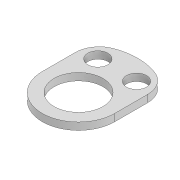
# Autodesk Inventor part: Sujeción mangueras
Saved by Autodesk Inventor 2022 (Build 260153000, 153)
## iProperties
Created: 2022-10-26
Part Number: Sujeción mangueras
Material: Generic
Document SubType Name: Modeling
Designer: ADMIN
Density: 1 g/cm^3
Appearance: Default
Author: ADMIN
## iProperties of the stored document Sujeción mangueras_3DPrint.ipt
Created: 2022-10-26
Part Number: Sujeción mangueras_3DPrint
Material: Generic
Document SubType Name: Modeling
Designer: ADMIN
Density: 1 g/cm^3
Appearance: Default
Author: ADMIN
Autodesk Inventor part; units mm, degrees
ref_plane "YZ Plane" through (0, 0, 0) normal (1, 0, 0) x (0, 1, 0)
ref_plane "XZ Plane" through (0, 0, 0) normal (0, 1, 0) x (-1, 0, 0)
ref_plane "XY Plane" through (0, 0, 0) normal (0, 0, 1) x (1, 0, 0)
sketch "Sketch1" plane through (0, 0, 0) normal (0, 1, 0) x (-1, 0, 0)
  circle A0 centre (0, 0) radius 10.1
  circle A1 centre (8, -16) radius 4.15
  circle A2 centre (-8, -16) radius 4.15
  circle A3 centre (0, 0) radius 24.4957
  line L0 (15, 0) -> (15, -19.3659)
  line L1 (-15, 0) -> (-15, -19.3659)
  arc A4 (15, 0) -> (-15, 0) centre (0, 0) ccw
  arc A5 (-9.0276, -11.9792) -> (-4.1668, -14.4096) centre (0, 0) ccw
  dimension "d0" = 20.2
  dimension "d1" = 8.3
  dimension "d2" = 8.3
  dimension "d3" = 16
  dimension "d4" = 16
  dimension "d5" = 16
  dimension "d6" = 8
  constraints: 8 point on circle, 6 centre point, 4 end point, 3 coincident, 1 parallel, 1 vertical
  measures "d0" diameter of A0
  measures "d1" diameter of A1
  measures "d2" diameter of A2
  measures "d3" distance of A2.centre A1.centre
  measures "d4" vertical distance of A0.centre A1.centre
  measures "d5" vertical distance of point (0, 0) A2.centre
  measures "d6" horizontal distance of point (0, 0) A1.centre
extrude "Extrusion1" add sketch "Sketch1" along normal blind 3 contours L1 A4 L0 A3 picked at (13.8916, -11.1458)
fillet "Fillet1" radius 10 2 edges at (15, 1.5, -19.3659) (-15, 1.5, -19.3659)
equation "\"d2\" = d1"
body "Solid1"
